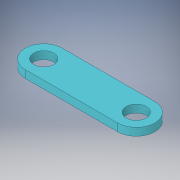
# Autodesk Inventor part: Middle_leg_b
Saved by Autodesk Inventor 2017 (Build 210142000, 142)
## iProperties
Created: 2016-06-08
Part Number: Middle_leg_b
Material: Generic
Document SubType Name: Modeling
Designer: alex-
Density: 1 g/cm^3
Appearance: Cadet Blue
Author: alex-
Autodesk Inventor part; units mm, degrees
ref_plane "YZ Plane" through (0, 0, 0) normal (1, 0, 0) x (0, 1, 0)
ref_plane "XZ Plane" through (0, 0, 0) normal (0, 1, 0) x (-1, 0, 0)
ref_plane "XY Plane" through (0, 0, 0) normal (0, 0, 1) x (1, 0, 0)
sketch "Sketch1" plane through (0, 0, 0) normal (0, 1, 0) x (-1, 0, 0)
  circle A0 centre (30, 0) radius 12
  circle A1 centre (-30, 0) radius 12
  line L0 (-30, 12) -> (30, 12)
  line L1 (-30, -12) -> (30, -12)
  circle A2 centre (30, 0) radius 6.5
  circle A3 centre (-30, 0) radius 6.5
  point P0 (0, 0)
  point P1 (0, 12)
  dimension "d0" = 60
  dimension "d1" = 24
  dimension "d2" = 13
  constraints: 4 centre point, 4 end point, 4 point on circle, 4 tangent, 2 coincident, 2 horizontal alignment, 1 equal radius, 1 midpoint, 1 parallel, 1 vertical alignment
  measures "d0" distance of A1.centre A0.centre
  measures "d1" diameter of A0
  measures "d2" diameter of A2
extrude "Extrusion1" add sketch "Sketch1" along normal blind 5
equation "\"d1\" = sa_diameter"
equation "\"d2\" = bb_outer_diameter"
equation "\"d3\" = b_mat_thickness"
equation "\"sa_diameter\" = 24"
equation "\"bb_outer_diameter\" = 13"
equation "\"b_mat_thickness\" = 5"
body "Solid1"
